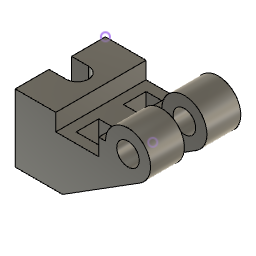
drawing_11 v1 (Autodesk Fusion 360 design; units mm, degrees)
Autodesk Fusion 360 part; units mm, degrees
note: some values were not read from the file. Set by a fixed rule: which sketch regions a step uses.
sketch "Sketch1" plane through (0, 0, 0) normal (0, 0, 1) x (1, 0, 0)
  line L0 (0, 0) -> (21, 0)
  line L1 (21, 0) -> (0, 0)
  line L2 (0, 0) -> (-21, 0)
  line L3 (-21, 0) -> (-21, -40)
  line L4 (21, 0) -> (21, 40)
  line L5 (21, 40) -> (-21, 40)
  line L6 (-21, 40) -> (-21, -40)
  line L7 (-21, -40) -> (21, -40)
  line L8 (21, -40) -> (21, 40)
  dimension "d1" = 21
  dimension "d2" = 21
  dimension "d3" = 40
  dimension "d4" = 40
  constraint coincident L0.start L1.end
  constraint horizontal L0
  constraint parallel L0 L2
  constraint perpendicular L2 L3
  constraint perpendicular L0 L4
  constraint horizontal L5
  constraint vertical L6
  constraint horizontal L7
  constraint vertical L8
  measures "d1" distance of L0.start L0.end
  measures "d2" distance of L0.start L2.end
  measures "d3" distance of L2.end L3.end
  measures "d4" distance of L0.end L4.end
extrude "Extrude1" add sketch "Sketch1" along normal blind 60 makes body 1
sketch "Sketch2" plane through (0, -40, 0) normal (0, -1, 0) x (1, 0, 0)
  line L0 (-21, 0) -> (21, 0)
  line L1 (21, 0) -> (21, 60)
  line L2 (21, 60) -> (-21, 60)
  line L3 (-21, 60) -> (-21, 0)
  line L4 (-21, 60) -> (99, 60)
  line L5 (21, 0) -> (99, 60)
  dimension "d7" = 120
  constraint coincident L2.end L3.start
  constraint perpendicular L3 L4
  constraint coincident L0.end L1.start
  measures "d7" distance of L2.end L4.end
extrude "Extrude2" add sketch "Sketch2" against normal blind 80 contours L1 L4 L5 bodies 1
sketch "Sketch3" plane through (0, 40, 0) normal (0, 1, 0) x (-1, 0, 0)
  line L0 (-21, 0) -> (21, 0)
  line L1 (21, 0) -> (21, 60)
sketch "Sketch4" plane through (0, 0, 60) normal (0, 0, 1) x (-1, 0, 0)
  line L0 (-99, -40) -> (21, -40)
  line L1 (21, -40) -> (21, 40)
  line L2 (21, 40) -> (-99, 40)
  line L3 (-99, 40) -> (-99, -40)
  line L4 (-79, 40) -> (6, 40)
  circle A0 centre (6, 0) radius 10
  point P0 (21, 0)
  point P1 (6, 0)
  dimension "d13" = 85
  dimension "d14" = 20
  constraint midpoint L1 P0
  constraint parallel L2 L4
  constraint coincident P1 A0.centre
  measures "d13" distance of L4.start L4.end
  measures "d14" diameter of A0
extrude "Extrude3" cut sketch "Sketch4" against normal blind 234 contours A0 bodies 1
sketch "Sketch5" plane through (0, 0, 60) normal (0, 0, 1) x (-1, 0, 0)
  circle A0 centre (6, 0) radius 10
  line L0 (-99, -40) -> (21, -40)
  line L1 (21, -40) -> (21, 40)
  line L2 (21, 40) -> (-99, 40)
  line L3 (-99, 40) -> (-99, -40)
  circle A1 centre (6, 0) radius 10
  line L4 (6, -10) -> (6, 10)
  line L5 (6, -10) -> (21, -10)
  line L6 (6, 10) -> (21, 10)
  constraint concentric A0 A1
  constraint coincident A0 L4.start
  constraint coincident A0 L4.end
  constraint parallel L1 L4
  constraint coincident L1 L5.end
  constraint tangent A0 L5
  constraint perpendicular L1 L5
  constraint coincident L1 L6.end
  constraint perpendicular L1 L6
extrude "Extrude4" cut sketch "Sketch5" against normal blind 30 contours A0 L1 A1 L5 L6 bodies 1
sketch "Sketch6" plane through (0, 0, 60) normal (0, 0, 1) x (-1, 0, 0)
  line L0 (21, -10) -> (6, -10)
  arc A0 (6, 10) -> (6, -10) centre (6, 0) ccw
  line L1 (6, 10) -> (21, 10)
  line L2 (21, 10) -> (21, 40)
  line L3 (21, 40) -> (-99, 40)
  line L4 (-99, 40) -> (-99, -40)
  line L5 (-99, -40) -> (21, -40)
  line L6 (21, -40) -> (21, -10)
  line L7 (21, 40) -> (-79, 40)
  line L8 (-79, 40) -> (-34, 40)
  line L9 (-99, 0) -> (-99, 21)
  line L10 (-99, 0) -> (-99, -21)
  line L11 (-24, -31) -> (-44, -31)
  line L12 (-44, -31) -> (-44, -11)
  line L13 (-44, -11) -> (-24, -11)
  line L14 (-24, -11) -> (-24, -31)
  line L15 (-24, -31) -> (-44, -11) construction
  line L16 (-44, -31) -> (-24, -11) construction
  line L17 (-44, 11) -> (-24, 11)
  line L18 (-24, 11) -> (-24, 31)
  line L19 (-24, 31) -> (-44, 31)
  line L20 (-44, 31) -> (-44, 11)
  line L21 (-44, 11) -> (-24, 31) construction
  line L22 (-24, 11) -> (-44, 31) construction
  point P0 (-99, 0)
  point P1 (-34, 21)
  point P2 (-34, -21)
  point P3 (-34, -21)
  point P4 (-34, 21)
  dimension "d23" = 20
  dimension "d24" = 20
  dimension "d25" = 20
  dimension "d26" = 20
  constraint coincident L2.end L3.start
  constraint perpendicular L2 L7
  constraint parallel L3 L8
  constraint coincident P0 L9.start
  constraint vertical L9
  constraint parallel L4 L10
  constraint horizontal L11
  constraint perpendicular L11 L12
  constraint parallel L11 L13
  constraint parallel L12 L14
  constraint coincident L15 P3
  constraint coincident L16 P3
  constraint coincident P3 P2
  constraint horizontal L17
  constraint perpendicular L17 L18
  constraint parallel L17 L19
  constraint parallel L18 L20
  constraint coincident L21 P4
  constraint coincident L22 P4
  constraint coincident P4 P1
  measures "d23" distance of L12.end L13.end
  measures "d24" distance of L11.end L12.end
  measures "d25" distance of L18.end L19.end
  measures "d26" distance of L17.end L18.end
sketch "Sketch9" plane through (0, 0, 60) normal (0, 0, 1) x (-1, 0, 0)
  line L0 (21, -10) -> (6, -10)
  arc A0 (6, 10) -> (6, -10) centre (6, 0) ccw
  line L1 (6, 10) -> (21, 10)
  line L2 (21, 10) -> (21, 40)
  line L3 (21, 40) -> (-99, 40)
  line L4 (-99, 40) -> (-99, -40)
  line L5 (-99, -40) -> (21, -40)
  line L6 (21, -40) -> (21, -10)
  line L7 (-99, 40) -> (-135, 40)
  line L8 (-135, 40) -> (-135, -40)
  line L9 (-135, -40) -> (-99, -40)
  line L10 (-99, -40) -> (-99, 40)
  constraint horizontal L7
  constraint vertical L8
  constraint horizontal L9
  constraint vertical L10
  constraint coincident L3.end L4.start
extrude "Extrude7" add sketch "Sketch9" against normal blind 60 separate body contours L4 L7 L8 L9 L10 makes body 2
extrude "Extrude8" add 1 faces at (99, -13.3333, 40) along direction (-1, 0, 0) blind 85 on bodies 2 bodies 2 1
extrude "Extrude5" cut sketch "Sketch6" against normal blind 75 contours L11 L12 L13 L14 | L17 L18 L19 L20 bodies 2
sketch "Sketch7" plane through (0, 0, 60) normal (0, 0, 1) x (-1, 0, 0)
  line L0 (-44, -31) -> (-44, -11)
  line L1 (-44, -11) -> (-24, -11)
  line L2 (-24, -11) -> (-24, -31)
  line L3 (-24, -31) -> (-44, -31)
  line L4 (-24, 11) -> (-44, 11)
  line L5 (-44, 11) -> (-44, 31)
  line L6 (-44, 31) -> (-24, 31)
  line L7 (-24, 31) -> (-24, 11)
  line L8 (21, -10) -> (6, -10)
  arc A0 (6, 10) -> (6, -10) centre (6, 0) ccw
  line L9 (6, 10) -> (21, 10)
  line L10 (21, 10) -> (21, 40)
  line L11 (21, 40) -> (-135, 40)
  line L12 (-135, -40) -> (21, -40)
  line L13 (21, -40) -> (21, -10)
  line L14 (-79, 40) -> (-34, 40)
  line L15 (-34, 40) -> (-53, 40)
  line L16 (-34, 40) -> (-15, 40)
  line L17 (-15, 40) -> (-53, 40)
  line L18 (-53, 40) -> (-53, -40)
  line L19 (-53, -40) -> (-15, -40)
  line L20 (-15, -40) -> (-15, 40)
  line L21 (-135, 40) -> (-135, -40)
  dimension "d30" = 45
  constraint parallel L11 L15
  constraint parallel L11 L16
  constraint horizontal L17
  constraint vertical L18
  constraint horizontal L19
  constraint vertical L20
  constraint coincident L12 L18.end
  measures "d30" distance of L14.start L14.end
extrude "Extrude6" cut sketch "Sketch7" against normal blind 15 contours L11 L12 L14 L15 L16 L17 L18 L19 L20 bodies 2
sketch "Sketch10" plane through (0, -40, 0) normal (0, -1, 0) x (1, 0, 0)
  line L0 (15, 45) -> (15, 60)
  line L1 (15, 60) -> (-21, 60)
  line L2 (-21, 60) -> (-21, 0)
  line L3 (-21, 0) -> (135, 0)
  line L4 (135, 0) -> (135, 60)
  line L5 (135, 60) -> (53, 60)
  line L6 (53, 60) -> (53, 45)
  line L7 (53, 45) -> (15, 45)
  circle A0 centre (79, 60) radius 20
  line L8 (-21, 0) -> (21, 0)
  line L9 (21, 0) -> (89.6293, 43.0584)
  dimension "d40" = 40
  dimension "d41" = 42
  constraint coincident L2.end L3.start
  constraint perpendicular L2 L8
  constraint coincident A0 L9.end
  constraint tangent A0 L9
  measures "d40" diameter of A0
  measures "d41" distance of L2.end L8.end
extrude "Extrude9" cut sketch "Sketch10" against normal blind 165 contours L3 L4 L5 A0 L9 bodies 2
sketch "Sketch11" plane through (0, -40, 0) normal (0, -1, 0) x (1, 0, 0)
  line L0 (21, 0) -> (89.6293, 43.0584)
  arc A0 (89.6293, 43.0584) -> (99, 60) centre (79, 60) ccw
  line L1 (99, 60) -> (53, 60)
  line L2 (53, 60) -> (53, 45)
  line L3 (53, 45) -> (15, 45)
  line L4 (15, 45) -> (15, 60)
  line L5 (15, 60) -> (-21, 60)
  line L6 (-21, 60) -> (-21, 0)
  line L7 (-21, 0) -> (21, 0)
  circle A1 centre (79, 60) radius 20
  dimension "d45" = 40
  measures "d45" diameter of A1
extrude "Extrude10" add sketch "Sketch11" against normal blind 80 contours A0 L1 A1 | L1 A1 bodies 2
sketch "Sketch12" plane through (0, -40, 0) normal (0, -1, 0) x (1, 0, 0)
  line L0 (59, 60) -> (53, 60)
  line L1 (53, 60) -> (53, 45)
  line L2 (53, 45) -> (15, 45)
  line L3 (15, 45) -> (15, 60)
  line L4 (15, 60) -> (-21, 60)
  line L5 (-21, 60) -> (-21, 0)
  line L6 (-21, 0) -> (21, 0)
  line L7 (21, 0) -> (89.6293, 43.0584)
  arc A0 (89.6293, 43.0584) -> (59, 60) centre (79, 60) ccw
  circle A1 centre (79, 60) radius 10
  dimension "d48" = 20
  constraint concentric A0 A1
  measures "d48" diameter of A1
extrude "Extrude11" cut sketch "Sketch12" against normal blind 180 contours A1 bodies 2
sketch "Sketch13" plane through (0, 0, 60) normal (0, 0, 1) x (-1, 0, 0)
  line L0 (-15, 40) -> (-15, -40)
  line L1 (-15, -40) -> (21, -40)
  line L2 (21, -40) -> (21, -10)
  line L3 (21, -10) -> (6, -10)
  arc A0 (6, 10) -> (6, -10) centre (6, 0) ccw
  line L4 (6, 10) -> (21, 10)
  line L5 (21, 10) -> (21, 40)
  line L6 (21, 40) -> (-15, 40)
  line L7 (-59, 0) -> (-59, -10)
  line L8 (-59, 0) -> (-59, 10)
  line L9 (-59, -10) -> (-105, -10)
  line L10 (-105, -10) -> (-105, 10)
  line L11 (-105, 10) -> (-59, 10)
  line L12 (-59, 10) -> (-59, -10)
  dimension "d52" = 10
  dimension "d53" = 10
  constraint horizontal L9
  constraint vertical L10
  constraint horizontal L11
  constraint vertical L12
  measures "d52" distance of L7.start L7.end
  measures "d53" distance of L7.start L8.end
extrude "Extrude12" cut sketch "Sketch13" along normal blind 50 and the other way blind 60 contours L7 L8 L9 L10 L11 L12 bodies 2
